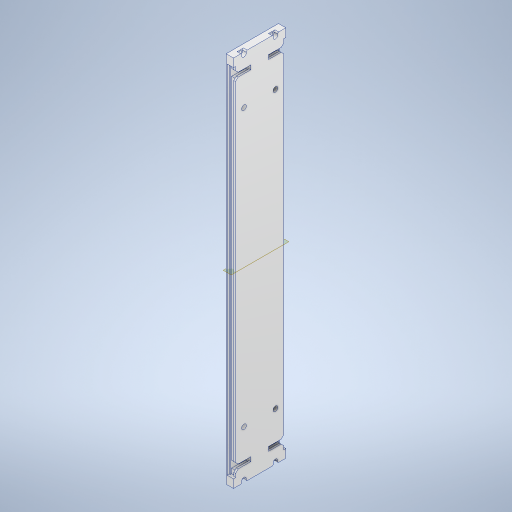
# Autodesk Inventor part: TopPaz
Saved by Autodesk Inventor 2024 (Build 280153000, 153)
## iProperties
Created: 2023-03-08
Part Number: TopPaz
Material: Алюминий 6061
Document SubType Name: Modeling
Designer: KirikDK
Density: 2.7 g/cm^3
Appearance: Алюминий — плоский
Mass: 2400.88 g
Surface Area: 1765.92 cm^2
Volume: 889.216 cm^3
Author: KirikDK
Autodesk Inventor part; units mm, degrees
ref_plane "YZ Plane" through (0, 0, 0) normal (1, 0, 0) x (0, 1, 0)
ref_plane "XZ Plane" through (0, 0, 0) normal (0, 1, 0) x (-1, 0, 0)
ref_plane "XY Plane" through (0, 0, 0) normal (0, 0, 1) x (1, 0, 0)
sketch "Эскиз1" plane through (0, 0, 0) normal (0, 1, 0) x (-1, 0, 0)
  line L0 (-6.0731, 25) -> (3.9269, 25)
  line L1 (-6.0731, -62) -> (-6.0731, 25)
  line L2 (3.9269, 31.5) -> (7.9269, 31.5)
  line L3 (7.9269, 31.5) -> (7.9269, -68.5)
  line L4 (3.9269, 25) -> (3.9269, 31.5)
  line L5 (-6.0731, 25) -> (-2.5731, 25)
  line L6 (-2.5731, 25) -> (-2.5731, 27.5)
  line L7 (-2.5731, 27.5) -> (-6.0731, 27.5)
  line L8 (-6.0731, 27.5) -> (-6.0731, 25)
  line L9 (3.9269, 27.5) -> (5.9269, 27.5)
  line L10 (5.9269, 27.5) -> (5.9269, 31.5)
  line L11 (5.9269, 31.5) -> (3.9269, 31.5)
  line L12 (3.9269, 31.5) -> (3.9269, 27.5)
  line L13 (7.9269, -18.5) -> (10, -18.5)
  line L14 (-6.0731, -62) -> (3.9269, -62)
  line L15 (3.9269, -68.5) -> (7.9269, -68.5)
  line L16 (3.9269, -62) -> (3.9269, -68.5)
  line L17 (-6.0731, -62) -> (-2.5731, -62)
  line L18 (-2.5731, -62) -> (-2.5731, -64.5)
  line L19 (-2.5731, -64.5) -> (-6.0731, -64.5)
  line L20 (-6.0731, -64.5) -> (-6.0731, -62)
  line L21 (3.9269, -64.5) -> (5.9269, -64.5)
  line L22 (5.9269, -64.5) -> (5.9269, -68.5)
  line L23 (5.9269, -68.5) -> (3.9269, -68.5)
  line L24 (3.9269, -68.5) -> (3.9269, -64.5)
  point P0 (0, 0)
  point P1 (-2.5731, 25)
  dimension "d0" = 14
  dimension "d1" = 6.5
  dimension "d2" = 6.5
  dimension "d3" = 2.5
  dimension "d4" = 4
  dimension "d5" = 2
  dimension "d6" = 100
  dimension "d7" = 50
  constraints: 50 end point, 10 symmetric about line, 5 horizontal, 5 parallel, 3 perpendicular, 2 midpoint, 2 point on line
  measures "d0" distance between parallel lines of L3 L1
  measures "d1" distance of L0.end L2.start
  measures "d2" distance between parallel lines of L4 L6
  measures "d3" distance of L7.end L0.start
  measures "d4" distance of L9.end L10.end
  measures "d5" distance of L10.end L11.end
  measures "d6" distance of L2.end L3.end
  measures "d7" distance between parallel lines of L2 L13
extrude "Выдавливание1" add sketch "Эскиз1" along normal blind 712 contours L8 L7 L6 L0 | L0 L4 L9 L10 L2 L3 L15 L22 L21 L16 L14 L1 | L14 L18 L19 L20
sketch "Эскиз5" plane through (-5.9269, 0, 31.5) normal (0, 0, 1) x (1, 0, 0)
  line L0 (-2, 0) -> (12, 0)
  line L1 (12, 0) -> (12, 16)
  line L2 (12, 16) -> (-2, 16)
  line L3 (-2, 16) -> (-2, 0)
  line L4 (-2, 0) -> (-2, 712) projected
  line L5 (12, 712) -> (8.5, 712) projected
  line L6 (12, 712) -> (-2, 712)
  line L7 (-2, 712) -> (-2, 696)
  line L8 (-2, 696) -> (12, 696)
  line L9 (12, 696) -> (12, 712)
  point P0 (5.9269, 0)
  dimension "d18" = 16
  dimension "d19" = 0
  dimension "d20" = 16
  constraints: 16 end point, 4 parallel, 2 horizontal, 2 perpendicular, 1 point on line
  measures "d18" distance of L0.end L1.end
  measures "d19" distance between parallel lines of L4 L3
  measures "d20" distance of L8.end L5.start
extrude "Выдавливание3" add sketch "Эскиз5" against normal blind 100
sketch "Эскиз6" plane through (-7.9269, 0, 31.5) normal (0, 0, 1) x (1, 0, 0)
  line L0 (14, 25.5) -> (4, 25.5)
  line L1 (14, 25.5) -> (10.5, 25.5)
  line L2 (10.5, 25.5) -> (10.5, 28)
  line L3 (10.5, 28) -> (14, 28)
  line L4 (14, 28) -> (14, 25.5)
  line L5 (4, 32) -> (0, 32)
  line L6 (2, 28) -> (2, 32)
  line L7 (2, 32) -> (4, 32)
  line L8 (4, 32) -> (4, 28)
  line L9 (4, 25.5) -> (4, 32)
  line L10 (4, 28) -> (2, 28)
  line L11 (14, 38.5) -> (4, 38.5)
  line L12 (14, 38.5) -> (10.5, 38.5)
  line L13 (10.5, 36) -> (14, 36)
  line L14 (14, 36) -> (14, 38.5)
  line L15 (10.5, 38.5) -> (10.5, 36)
  line L16 (4, 36) -> (2, 36)
  line L17 (2, 36) -> (2, 32)
  line L18 (4, 32) -> (4, 36)
  line L19 (4, 38.5) -> (4, 32)
  line L20 (14, 36) -> (14, 28)
  line L21 (14, 16) -> (14, 696) projected
  line L22 (14, 356) -> (16, 356)
  line L23 (0, 0) -> (14, 0) projected
  line L24 (14, 686.5) -> (4, 686.5)
  line L25 (14, 686.5) -> (10.5, 686.5)
  line L26 (10.5, 684) -> (14, 684)
  line L27 (14, 684) -> (14, 686.5)
  line L28 (10.5, 686.5) -> (10.5, 684)
  line L29 (4, 684) -> (2, 684)
  line L30 (4, 680) -> (0, 680)
  line L31 (2, 684) -> (2, 680)
  line L32 (2, 680) -> (4, 680)
  line L33 (4, 680) -> (4, 684)
  line L34 (4, 686.5) -> (4, 680)
  line L35 (14, 673.5) -> (4, 673.5)
  line L36 (14, 673.5) -> (10.5, 673.5)
  line L37 (10.5, 676) -> (14, 676)
  line L38 (14, 676) -> (14, 673.5)
  line L39 (10.5, 673.5) -> (10.5, 676)
  line L40 (4, 676) -> (2, 676)
  line L41 (2, 676) -> (2, 680)
  line L42 (4, 680) -> (4, 676)
  line L43 (4, 673.5) -> (4, 680)
  line L44 (14, 676) -> (14, 684)
  point P0 (7.9269, 0)
  dimension "d26" = 356
  constraints: 86 end point, 25 symmetric about line, 4 point on line, 1 collinear, 1 horizontal, 1 midpoint
  measures "d26" distance between parallel lines of L22 L23
extrude "Выдавливание4" cut sketch "Эскиз6" against normal blind 100 contours L0 L9 L8 L18 L19 L11 L15 L13 L20 L3 L2 | L37 L39 L35 L43 L42 L33 L34 L24 L28 L26 L21
chamfer "Фаска2" distance 4.99 angle 45 8 edges at (4.3231, 684, 27.5) (4.3231, 676, 27.5) (4.3231, 36, 27.5) (4.3231, 28, 27.5) (4.3231, 36, -64.5) (4.3231, 28, -64.5) (4.3231, 684, -64.5) (4.3231, 676, -64.5)
sketch "Эскиз7" plane through (6.0731, 40.99, 27.5) normal (1, 0, 0) x (0, 0, -1)
  circle A0 centre (76, 51.01) radius 2.5
  circle A1 centre (16, 51.01) radius 2.5
  line L0 (-4, -24.99) -> (-4, 655.01) projected
  line L1 (96, -24.99) -> (96, 655.01) projected
  line L2 (-4, -40.99) -> (96, -40.99) projected
  circle A2 centre (76, -36.99) radius 2.5
  circle A3 centre (16, -36.99) radius 2.5
  point P0 (27.5, -40.99)
  dimension "d32" = 5
  dimension "d33" = 20
  dimension "d34" = 20
  dimension "d35" = 5
  dimension "d36" = 92
  dimension "d37" = 92
  dimension "d38" = 5
  dimension "d39" = 5
  dimension "d40" = 4
  dimension "d41" = 4
  constraints: 4 centre point
  measures "d32" diameter of A0
  measures "d33" distance from line of A1.centre L0
  measures "d34" distance from line of A0.centre L1
  measures "d35" diameter of A1
  measures "d36" distance from line of L2 A0.centre
  measures "d37" distance from line of L2 A1.centre
  measures "d38" diameter of A2
  measures "d39" diameter of A3
  measures "d40" distance from line of L2 A3.centre
  measures "d41" distance from line of L2 A2.centre
ref_plane "РабПлоскость1" through (0, 356, 0) normal (0, -1, 0) x (1, 0, 0)
hole "Отверстие1" at (6.0731, 4, 11.5) at (6.0731, 4, -48.5) at (6.0731, 92, -48.5) at (6.0731, 92, 11.5) direction (-1, 0, 0) diameter 5 end through all counterbore diameter 9 counterbore depth 7
mirror "Зеркальное отражение1" about plane through (0, 356, 0) normal (0, -1, 0) of "Отверстие1"
fillet "Сопряжение2" radius 2 8 edges at (2.5731, 0, -50.5616) (2.5731, 0, -46.4384) (2.5731, 0, 9.4384) (2.5731, 0, 13.5616) (2.5731, 712, -50.5616) (2.5731, 712, -46.4384) (2.5731, 712, 9.4384) (2.5731, 712, 13.5616)
sketch "Sketch8" plane through (6.0731, 40.99, 27.5) normal (1, 0, 0) x (0, 0, -1)
  line L0 (96, -40.99) -> (-4, -40.99) projected
  circle A0 centre (46, -40.99) radius 17
  line L1 (96, 671.01) -> (-4, 671.01) projected
  line L2 (29, -40.99) -> (63, -40.99)
  line L3 (63, -40.99) -> (63, 671.01)
  line L4 (63, 671.01) -> (29, 671.01)
  line L5 (29, 671.01) -> (29, -40.99)
  point P0 (27.5, -40.99)
  dimension "d51" = 34
  constraints: 8 end point, 2 parallel, 2 point on line, 1 horizontal, 1 midpoint, 1 perpendicular, 3 other
extrude "Extrusion5" add sketch "Sketch8" against normal blind 10 contours A0 L5 L1 L3
